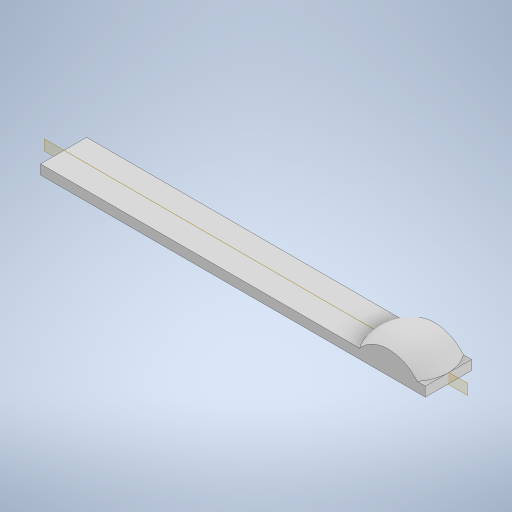
# Autodesk Inventor part: strain sensor silicone
Saved by Autodesk Inventor 2024.2 (Build 282272000, 272)
## iProperties
Created: 2025-02-11
Part Number: strain sensor silicone
Material: Generic
Document SubType Name: Modeling
Designer: Tom
Density: 1 g/cm^3
Appearance: Default
Author: Tom
Autodesk Inventor part; units mm, degrees
ref_plane "YZ Plane" through (0, 0, 0) normal (1, 0, 0) x (0, 1, 0)
ref_plane "XZ Plane" through (0, 0, 0) normal (0, 1, 0) x (-1, 0, 0)
ref_plane "XY Plane" through (0, 0, 0) normal (0, 0, 1) x (1, 0, 0)
sketch "Sketch1" plane through (0, 0, 0) normal (0, 1, 0) x (-1, 0, 0)
  line L0 (0, 0) -> (63.5, 0)
  line L1 (63.5, 0) -> (63.5, -7.62)
  line L2 (63.5, -7.62) -> (0, -7.62)
  line L3 (0, -7.62) -> (0, 0)
  dimension "d0" = 7.62
  dimension "d1" = 63.5
  constraints: 8 end point, 2 parallel, 1 horizontal, 1 perpendicular
  measures "d0" distance of L2.end L0.start
  measures "d1" distance of L1.end L2.end
extrude "Extrusion1" add sketch "Sketch1" along normal blind 1.5875
ref_plane "Work Plane1" through (-63.5, 0, -3.81) normal (0, 0, 1) x (1, 0, 0)
sketch "Sketch2" plane through (-63.5, 0, -3.81) normal (0, 0, 1) x (1, 0, 0)
  line L0 (61.7107, 1.5875) -> (61.7107, -0.5013)
  line L1 (61.7619, 1.5875) -> (63.5, 1.5875)
  arc A0 (63.5, 1.5875) -> (57.4176, 4.8744) centre (57.4576, -2.3227) ccw
  line L2 (57.4176, 4.8744) -> (57.4176, 1.5875)
  line L3 (57.4176, 1.5875) -> (63.5, 1.5875)
  point P0 (63.5, 0)
  constraints: 8 end point, 2 point on circle, 2 vertical, 1 centre point, 1 perpendicular
revolve "Revolution1" add sketch "Sketch2" angle 360 about axis through (-6.0824, 4.8744, -3.81) along (0, -1, 0)
sketch "Sketch3" plane through (0, 0, 0) normal (1, 0, 0) x (0, 0, -1)
  line L0 (0, 0) -> (-3.2276, 0)
  line L1 (-3.2276, 0) -> (-3.2276, 6.1227)
  line L2 (-3.2276, 6.1227) -> (0, 6.1227)
  line L3 (0, 6.1227) -> (0, 0)
  line L4 (7.6049, 0) -> (10.3754, 0)
  line L5 (10.3754, 0) -> (10.3754, 5.4855)
  line L6 (10.3754, 5.4855) -> (7.6049, 5.4855)
  line L7 (7.6049, 5.4855) -> (7.6049, 0)
  constraints: 16 end point, 4 parallel, 2 horizontal, 2 perpendicular, 1 point on line
extrude "Extrusion2" cut sketch "Sketch3" against normal through all
body "Solid1"
